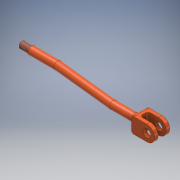
# Autodesk Inventor part: eccentric rod
Saved by Autodesk Inventor 2017 (Build 210142000, 142)
## iProperties
Created: 2018-11-18
Part Number: eccentric rod
Material: Steel, Alloy
Document SubType Name: Modeling
Designer: Arman Grewal
Density: 7.73 g/cm^3
Appearance: Smooth - Light Orange
Author: Arman Grewal
Autodesk Inventor part; units mm, degrees
ref_plane "XZ Plane" through (0, 0, 0) normal (0, 1, 0) x (-1, 0, 0)
ref_plane "XY Plane" through (0, 0, 0) normal (0, 0, 1) x (1, 0, 0)
sketch "Sketch1" plane through (0, 0, 0) normal (1, 0, 0) x (0, 1, 0)
  circle A0 centre (0, 0) radius 1.5
  dimension "d0" = 3
  constraints: 1 centre point, 1 coincident
  measures "d0" diameter of A0
ref_plane "Work Plane1" through (24, 0, 0) normal (1, 0, 0) x (0, 1, 0)
sketch "Sketch2" plane through (24, 0, 0) normal (1, 0, 0) x (0, 1, 0)
  line L0 (0, 0) -> (-2.5, 0) construction
  circle A0 centre (-2.5, 0) radius 1.5
  dimension "d2" = 2.5
  dimension "d3" = 3
  constraints: 2 end point, 1 centre point, 1 coincident, 1 horizontal
  measures "d2" distance of L0.start L0.end
  measures "d3" diameter of A0
loft "Loft1" add profiles "Sketch1", "Sketch2"
sketch "Sketch3" plane through (0, 0, 0) normal (-1, 0, 0) x (0, 0, 1)
  circle A0 centre (0, 0) radius 1.5 projected
  circle A1 centre (0, 0) radius 1.5
  dimension "d8" = 3
  constraints: 1 centre point, 1 coincident
  measures "d8" diameter of A1
extrude "Extrusion1" add sketch "Sketch3" along normal blind 10
sketch "Sketch4" plane through (-10, 0, 0) normal (-1, 0, 0) x (0, 0, 1)
  circle A0 centre (0, 0) radius 1.25
  dimension "d11" = 2.5
  constraints: 1 centre point, 1 coincident
  measures "d11" diameter of A0
extrude "Extrusion2" add sketch "Sketch4" along normal blind 4
thread "Thread1" size "M2.5x0.45" class "6g" standard "ANSI Metric M Profile" full length
chamfer "Chamfer1" distance 0.25 angle 45 1 edges at (-14, 0, -1.25)
sketch "Sketch5" plane through (24, -2.5, 0) normal (1, 0, 0) x (0, 0, -1)
  circle A0 centre (0, 0) radius 1.5
  circle A1 centre (0, 0) radius 1.5 projected
  line L0 (-1.4999, -0.019) -> (-1.4999, 7.557) construction
  point P0 (0, 2.5)
  dimension "d16" = 3
  dimension "d17" = 2.5
  dimension "d18" = 1.4999
  constraints: 2 end point, 1 vertical, 5 other
  measures "d17" distance of point (0, 2.5) point (0, 0)
  measures "d18" distance from line of point (0, 0) L0
extrude "Extrusion3" add sketch "Sketch5" along normal blind 10
sketch "Sketch6" plane through (34, -2.5, 0) normal (1, 0, 0) x (0, 0, -1)
  line L0 (-3, 3) -> (3, 3)
  line L1 (3, 3) -> (3, -3)
  line L2 (3, -3) -> (-3, -3)
  line L3 (-3, -3) -> (-3, 3)
  line L4 (-3, 3) -> (3, -3) construction
  line L5 (3, 3) -> (-3, -3) construction
  point P0 (0, 2.5)
  point P1 (0, 0)
  dimension "d24" = 6
  dimension "d25" = 6
  dimension "d26" = 3
  dimension "d27" = 0.5
  constraints: 12 end point, 2 midpoint, 2 parallel, 1 horizontal, 1 perpendicular
  measures "d24" distance of L1.end L2.end
  measures "d25" distance of L0.end L1.end
  measures "d26" distance from line of point (0, 2.5) L1
  measures "d27" distance from line of point (0, 2.5) L0
extrude "Extrusion4" add sketch "Sketch6" along normal blind 2
sketch "Sketch7" plane through (34, 0.5, 3) normal (0, 1, 0) x (1, 0, 0)
  line L0 (0, 0) -> (0, 6) projected
  line L1 (0, 6) -> (0, 0)
  line L2 (0, 6) -> (6, 6)
  line L3 (0, 0) -> (6, 0)
  circle A0 centre (6, 3) radius 1.5
  arc A1 (6, 0) -> (6, 6) centre (6, 3) ccw
  point P0 (-34, 3)
  dimension "d30" = 6
  dimension "d32" = 3
  constraints: 6 end point, 2 centre point, 2 point on circle, 2 tangent, 1 collinear, 1 concentric, 1 horizontal, 1 perpendicular
  measures "d30" distance of L0.end L2.end
  measures "d32" diameter of A0
extrude "Extrusion5" add sketch "Sketch7" against normal blind 1.5
sketch "Sketch8" plane through (34, -5.5, -3) normal (0, -1, 0) x (1, 0, 0)
  line L0 (0, 0) -> (0, 6) projected
  line L1 (0, 6) -> (0, 0)
  arc A0 (6, 0) -> (6, 6) centre (6, 3) ccw projected
  line L2 (0, 6) -> (6, 6)
  line L3 (0, 6) -> (6, 6) construction
  line L4 (0, 0) -> (6, 0) projected
  line L5 (0, 0) -> (6, 0)
  circle A1 centre (6, 3) radius 1.5
  line L6 (0, 6) -> (6, 6) projected
  arc A2 (6, 0) -> (6, 6) centre (6, 3) ccw
  point P0 (-34, 3)
  dimension "d35" = 6
  dimension "d36" = 0
  dimension "d37" = 3
  constraints: 8 end point, 3 collinear, 2 centre point, 2 horizontal, 2 point on circle, 2 tangent, 1 coincident, 1 vertical alignment
  measures "d35" distance of L0.end L2.end
  measures "d36" distance between parallel lines of L2 L3
  measures "d37" diameter of A1
extrude "Extrusion6" add sketch "Sketch8" against normal blind 1.5
fillet "Fillet2" radius 1.5 1 edges at (34, -2.5, 1.5)
fillet "Fillet4" radius 1 1 edges at (36, -1, 0)
fillet "Fillet5" radius 1 1 edges at (36, -4, 0)
fillet "Fillet6" radius 1 2 edges at (34, -2.5, 3) (34, -2.5, -3)
fillet "Fillet7" radius 0.1 28 edges at (38.5, -1, 3) (36.2929, -1.2929, 3) (36, -2.5, 3) (36.2929, -3.7071, 3) (38.5, -4, 3) (43, -4, 0) (38.5, -4, -3) (36.2929, -3.7071, -3) (36, -2.5, -3) (36.2929, -1.2929, -3) (38.5, -1, -3) (43, -1, 0) (38.5, 0.5, 0) (38.5, -4, 0) (38.5, -5.5, 0) (38.5, -1, 0) (43, 0.5, 0) (37.5, 0.5, -3) (34.2929, 0.5, -2.7071) (34, 0.5, 0) (34.2929, 0.5, 2.7071) (37.5, 0.5, 3) (37.5, -5.5, 3) (34.2929, -5.5, 2.7071) (34, -5.5, 0) (34.2929, -5.5, -2.7071) (37.5, -5.5, -3) (43, -5.5, 0)
body "Solid1"
